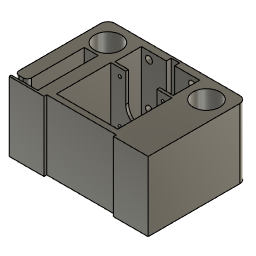
maturita1 v13 asi final (Autodesk Fusion 360 design; units mm, degrees)
Autodesk Fusion 360 part; units mm, degrees
note: some values were not read from the file. Chosen so that the rebuilt part matches the saved one: that a step has no effect. Set by a fixed rule: which sketch regions a step uses.
sketch "Sketch1" plane through (0, 0, 0) normal (0, 0, 1) x (1, 0, 0)
  line L0 (0, 0) -> (25, 0)
  line L1 (25, 0) -> (25, 2)
  line L2 (25, 2) -> (75, 2)
  line L3 (75, 2) -> (75, 0)
  line L4 (75, 0) -> (100, 0)
  line L5 (100, 0) -> (100, 71)
  line L6 (100, 71) -> (0, 71)
  line L7 (0, 71) -> (0, 0)
  dimension "d1" = 50
  dimension "d2" = 25
  dimension "d3" = 71
  constraint coincident L0.start L7.end
  constraint horizontal L0
  constraint perpendicular L0 L1
  constraint perpendicular L1 L2
  constraint perpendicular L2 L3
  constraint perpendicular L3 L4
  constraint perpendicular L4 L5
  constraint perpendicular L5 L6
  constraint perpendicular L0 L7
  measures "d1" distance of L1.end L2.end
  measures "d2" distance of L3.end L4.end
  measures "d3" distance of L4.end L5.end
extrude "Extrude1" add sketch "Sketch1" along normal blind 50
sketch "Sketch2" plane through (0, 0, 50) normal (0, 0, 1) x (-1, 0, 0)
  line L0 (0, -71) -> (0, 0)
  line L1 (0, 0) -> (-25, 0)
  line L2 (-25, 0) -> (-25, -2)
  line L3 (-25, -2) -> (-75, -2)
  line L4 (-75, -2) -> (-75, 0)
  line L5 (-75, 0) -> (-100, 0)
  line L6 (-100, 0) -> (-100, -71)
  line L7 (-100, -71) -> (0, -71)
  line L8 (0, -71) -> (-14.5, -71)
  line L9 (-14.5, -71) -> (-14.5, -56.5)
  circle A0 centre (-14.5, -56.5) radius 9.6
  line L10 (-14.5, -56.5) -> (-85.5, -56.5)
  circle A1 centre (-85.5, -56.5) radius 9.6
  dimension "d6" = 14.5
  dimension "d7" = 14.5
  dimension "d8" = 19.2
  dimension "d9" = 71
  dimension "d10" = 19.2
  constraint coincident L0.start L7.end
  constraint perpendicular L0 L8
  constraint perpendicular L7 L9
  constraint coincident L9.end A0.centre
  constraint perpendicular L9 L10
  constraint coincident L10.end A1.centre
  measures "d6" distance of L0.start L8.end
  measures "d7" distance of L8.end L9.end
  measures "d8" diameter of A0
  measures "d9" distance of L9.end L10.end
  measures "d10" diameter of A1
extrude "Extrude2" cut sketch "Sketch2" against normal up to surface (50 mm away) contours L9 A0 L10 | L9 A0 L10 | A1
fillet "Fillet1" radius 5 2 edges at (100, 71, 25) (0, 71, 25)
sketch "Sketch3" plane through (0, 0, 50) normal (0, 0, 1) x (-1, 0, 0)
  arc A0 (-5, -71) -> (0, -66) centre (-5, -66) ccw
  line L0 (0, -66) -> (0, 0)
  line L1 (0, 0) -> (-25, 0)
  line L2 (-25, 0) -> (-25, -2)
  line L3 (-25, -2) -> (-75, -2)
  line L4 (-75, -2) -> (-75, 0)
  line L5 (-75, 0) -> (-100, 0)
  line L6 (-100, 0) -> (-100, -66)
  arc A1 (-100, -66) -> (-95, -71) centre (-95, -66) ccw
  line L7 (-95, -71) -> (-5, -71)
  circle A2 centre (-14.5, -56.5) radius 9.6
  circle A3 centre (-85.5, -56.5) radius 9.6
  line L8 (-14.5, -66.1) -> (-29, -66.1)
  line L9 (-29, -66.1) -> (-71, -66.1)
  line L10 (-71, -66.1) -> (-71, -47.1)
  line L11 (-71, -47.1) -> (-29, -47.1)
  line L12 (-29, -47.1) -> (-29, -66.1)
  dimension "d22" = 42
  dimension "d23" = 19
  constraint coincident A2 L8.start
  constraint tangent A2 L8
  constraint horizontal L9
  constraint vertical L10
  constraint horizontal L11
  constraint vertical L12
  measures "d22" distance of L8.end L9.end
  measures "d23" distance of L8.end L11.end
extrude "Extrude4" [no effect]
extrude "Extrude5" cut sketch "Sketch3" against normal up to surface (50 mm away) contours L9 L10 L11 L12
sketch "Sketch5" plane through (0, 0, 50) normal (0, 0, 1) x (-1, 0, 0)
  line L0 (-29, -47.1) -> (-29, -66.1)
  line L1 (-29, -66.1) -> (-71, -66.1)
  line L2 (-71, -66.1) -> (-71, -47.1)
  line L3 (-71, -47.1) -> (-29, -47.1)
  arc A0 (-5, -71) -> (0, -66) centre (-5, -66) ccw
  line L4 (0, -66) -> (0, 0)
  line L5 (0, 0) -> (-25, 0)
  line L6 (-25, 0) -> (-25, -2)
  line L7 (-25, -2) -> (-75, -2)
  line L8 (-75, -2) -> (-75, 0)
  line L9 (-75, 0) -> (-100, 0)
  line L10 (-100, 0) -> (-100, -66)
  arc A1 (-100, -66) -> (-95, -71) centre (-95, -66) ccw
  line L11 (-95, -71) -> (-5, -71)
  circle A2 centre (-14.5, -56.5) radius 9.6
  circle A3 centre (-85.5, -56.5) radius 9.6
  line L12 (-50, -2) -> (-28, -2)
  line L13 (-28, -2) -> (-28, -45.1)
  line L14 (-28, -45.1) -> (-72, -45.1)
  line L15 (-72, -45.1) -> (-72, -6.1)
  line L16 (-72, -6.1) -> (-28, -6.1)
  line L17 (-28, -6.1) -> (-28, -45.1)
  line L18 (-50, -6.1) -> (-41, -6.1)
  line L19 (-41, -6.1) -> (-59, -6.1)
  line L20 (-59, -6.1) -> (-59, -18.1)
  line L21 (-59, -18.1) -> (-41, -18.1)
  line L22 (-41, -18.1) -> (-41, -6.1)
  line L23 (-28, -45.1) -> (-38.75, -45.1)
  line L24 (-38.75, -45.1) -> (-61.25, -45.1)
  line L25 (-61.25, -45.1) -> (-61.25, -47.1)
  line L26 (-61.25, -47.1) -> (-38.75, -47.1)
  line L27 (-38.75, -47.1) -> (-38.75, -45.1)
  dimension "d28" = 22
  dimension "d29" = 43.1
  dimension "d30" = 44
  dimension "d31" = 39
  dimension "d32" = 9
  dimension "d33" = 18
  dimension "d34" = 12
  dimension "d35" = 10.75
  dimension "d36" = 22.5
  constraint midpoint L7 L12.start
  constraint parallel L7 L12
  constraint perpendicular L3 L13
  constraint horizontal L14
  constraint vertical L15
  constraint horizontal L16
  constraint vertical L17
  constraint midpoint L16 L18.start
  constraint parallel L16 L18
  constraint horizontal L19
  constraint vertical L20
  constraint horizontal L21
  constraint vertical L22
  constraint perpendicular L17 L23
  constraint horizontal L24
  constraint vertical L25
  constraint horizontal L26
  constraint vertical L27
  measures "d28" distance of L12.start L12.end
  measures "d29" distance of L12.end L13.end
  measures "d30" distance of L13.end L14.end
  measures "d31" distance of L13.end L16.end
  measures "d32" distance of L18.start L18.end
  measures "d33" distance of L18.end L19.end
  measures "d34" distance of L18.end L21.end
  measures "d35" distance of L13.end L23.end
  measures "d36" distance of L23.end L24.end
extrude "Extrude6" cut sketch "Sketch5" against normal up to surface (50 mm away) contours L16 L18 L19 L20 L21 L22
extrude "Extrude7" cut sketch "Sketch5" against normal blind 42 contours L13 L14 L15 L16 L17 L20 L21 L22 L23 L24
extrude "Extrude8" cut sketch "Sketch5" against normal blind 32 contours L3 L14 L24 L25 L26 L27
fillet "Fillet2" radius 11.25 2 edges at (38.75, 46.1, 18) (61.25, 46.1, 18)
sketch "Sketch7" plane through (0, 45.1, 0) normal (0, -1, 0) x (1, 0, 0)
  line L0 (38.75, 29.25) -> (38.75, 50)
  line L1 (38.75, 50) -> (28, 50)
  line L2 (28, 50) -> (28, 8)
  line L3 (28, 8) -> (72, 8)
  line L4 (72, 8) -> (72, 50)
  line L5 (72, 50) -> (61.25, 50)
  line L6 (61.25, 50) -> (61.25, 29.25)
  arc A0 (38.75, 29.25) -> (61.25, 29.25) centre (50, 29.25) ccw
  line L7 (28, 8) -> (34.5, 8)
  line L8 (34.5, 8) -> (34.5, 13.5)
  circle A1 centre (34.5, 13.5) radius 1.1
  dimension "d48" = 6.5
  dimension "d49" = 5.5
  dimension "d50" = 2.2
  constraint coincident L2.end L3.start
  constraint perpendicular L2 L7
  constraint perpendicular L3 L8
  constraint coincident L8.end A1.centre
  measures "d48" distance of L2.end L7.end
  measures "d49" distance of L7.end L8.end
  measures "d50" diameter of A1
extrude "Extrude9" cut sketch "Sketch7" against normal up to surface (25.9 mm away) contours A1
pattern_linear "R-Pattern1" count 2 spacing 31 along (1, 0, 0) count 2 spacing 31 along (0, 0, 1) of "Extrude9"
sketch "Sketch8" plane through (0, 71, 0) normal (0, 1, 0) x (-1, 0, 0)
  circle A0 centre (-65.5, 44.5) radius 1.1
  circle A1 centre (-34.5, 44.5) radius 1.1
  circle A2 centre (-65.5, 13.5) radius 1.1
  circle A3 centre (-34.5, 13.5) radius 1.1
  line L0 (-5, 0) -> (-5, 50)
  line L1 (-5, 50) -> (-95, 50)
  line L2 (-95, 50) -> (-95, 0)
  line L3 (-95, 0) -> (-5, 0)
  circle A4 centre (-65.5, 44.5) radius 2.5
  dimension "d57" = 5
  constraint concentric A0 A4
  measures "d57" diameter of A4
extrude "Extrude10" cut sketch "Sketch8" against normal up to surface (4.9 mm away) contours A4
pattern_linear "R-Pattern2" count 2 spacing 31 along (-1, 0, 0) count 2 spacing 31 along (0, 0, -1) of "Extrude10"
sketch "Sketch9" plane through (0, 0, 50) normal (0, 0, 1) x (-1, 0, 0)
  line L0 (-38.75, -45.1) -> (-38.75, -47.1)
  line L1 (-38.75, -47.1) -> (-29, -47.1)
  line L2 (-29, -47.1) -> (-29, -66.1)
  line L3 (-29, -66.1) -> (-71, -66.1)
  line L4 (-71, -66.1) -> (-71, -47.1)
  line L5 (-71, -47.1) -> (-61.25, -47.1)
  line L6 (-61.25, -47.1) -> (-61.25, -45.1)
  line L7 (-61.25, -45.1) -> (-72, -45.1)
  line L8 (-72, -45.1) -> (-72, -6.1)
  line L9 (-72, -6.1) -> (-28, -6.1)
  line L10 (-28, -6.1) -> (-28, -45.1)
  line L11 (-28, -45.1) -> (-38.75, -45.1)
  circle A0 centre (-85.5, -56.5) radius 9.6
  circle A1 centre (-14.5, -56.5) radius 9.6
  arc A2 (-5, -71) -> (0, -66) centre (-5, -66) ccw
  line L12 (0, -66) -> (0, 0)
  line L13 (0, 0) -> (-25, 0)
  line L14 (-25, 0) -> (-25, -2)
  line L15 (-25, -2) -> (-75, -2)
  line L16 (-75, -2) -> (-75, 0)
  line L17 (-75, 0) -> (-100, 0)
  line L18 (-100, 0) -> (-100, -66)
  arc A3 (-100, -66) -> (-95, -71) centre (-95, -66) ccw
  line L19 (-95, -71) -> (-5, -71)
  line L20 (-50, -66.1) -> (-53, -66.1)
  line L21 (-53, -66.1) -> (-47, -66.1)
  line L22 (-47, -66.1) -> (-47, -69.6)
  line L23 (-47, -69.6) -> (-53, -69.6)
  line L24 (-53, -69.6) -> (-53, -66.1)
  dimension "d64" = 3
  dimension "d65" = 6
  dimension "d66" = 3.5
  constraint midpoint L3 L20.start
  constraint parallel L3 L20
  constraint horizontal L21
  constraint vertical L22
  constraint horizontal L23
  constraint vertical L24
  measures "d64" distance of L20.start L20.end
  measures "d65" distance of L20.end L21.end
  measures "d66" distance of L20.end L23.end
extrude "Extrude11" cut sketch "Sketch9" against normal blind 26.5 contours L3 L20 L21 L22 L23 L24
fillet "Fillet3" radius 3 2 edges at (53, 67.85, 23.5) (47, 67.85, 23.5)
sketch "Sketch10" plane through (0, 0, 50) normal (0, 0, 1) x (-1, 0, 0)
  line L0 (-53, -69.6) -> (-53, -66.1)
  line L1 (-53, -66.1) -> (-71, -66.1)
  line L2 (-71, -66.1) -> (-71, -47.1)
  line L3 (-71, -47.1) -> (-61.25, -47.1)
  line L4 (-61.25, -47.1) -> (-61.25, -45.1)
  line L5 (-61.25, -45.1) -> (-72, -45.1)
  line L6 (-72, -45.1) -> (-72, -6.1)
  line L7 (-72, -6.1) -> (-28, -6.1)
  line L8 (-28, -6.1) -> (-28, -45.1)
  line L9 (-28, -45.1) -> (-38.75, -45.1)
  line L10 (-38.75, -45.1) -> (-38.75, -47.1)
  line L11 (-38.75, -47.1) -> (-29, -47.1)
  line L12 (-29, -47.1) -> (-29, -66.1)
  line L13 (-29, -66.1) -> (-47, -66.1)
  line L14 (-47, -66.1) -> (-47, -69.6)
  line L15 (-47, -69.6) -> (-53, -69.6)
  circle A0 centre (-85.5, -56.5) radius 9.6
  circle A1 centre (-14.5, -56.5) radius 9.6
  arc A2 (-5, -71) -> (0, -66) centre (-5, -66) ccw
  line L16 (0, -66) -> (0, 0)
  line L17 (0, 0) -> (-25, 0)
  line L18 (-25, 0) -> (-25, -2)
  line L19 (-25, -2) -> (-75, -2)
  line L20 (-75, -2) -> (-75, 0)
  line L21 (-75, 0) -> (-100, 0)
  line L22 (-100, 0) -> (-100, -66)
  arc A3 (-100, -66) -> (-95, -71) centre (-95, -66) ccw
  line L23 (-95, -71) -> (-5, -71)
  line L24 (0, 0) -> (-9, 0)
  line L25 (-9, 0) -> (-9, -4)
  line L26 (-9, -4) -> (-19, -4)
  line L27 (-19, -4) -> (-19, -45)
  line L28 (-19, -45) -> (-9, -45)
  line L29 (-9, -45) -> (-9, -4)
  line L30 (-19, -4) -> (0, -4)
  line L31 (0, -4) -> (0, -1.5)
  line L32 (0, -1.5) -> (-19, -1.5)
  line L33 (-19, -1.5) -> (-19, -4)
  dimension "d71" = 9
  dimension "d72" = 4
  dimension "d73" = 10
  dimension "d74" = 41
  dimension "d75" = 19
  dimension "d76" = 2.5
  constraint coincident L16.end L17.start
  constraint perpendicular L8 L24
  constraint perpendicular L24 L25
  constraint horizontal L26
  constraint vertical L27
  constraint horizontal L28
  constraint vertical L29
  constraint horizontal L30
  constraint vertical L31
  constraint horizontal L32
  constraint vertical L33
  measures "d71" distance of L16.end L24.end
  measures "d72" distance of L24.end L25.end
  measures "d73" distance of L25.end L26.end
  measures "d74" distance of L25.end L28.end
  measures "d75" distance of L26.end L30.end
  measures "d76" distance of L26.end L32.end
extrude "Extrude12" cut sketch "Sketch10" against normal blind 16.5 contours L16 L25 L30 L31 L32 | L25 L26 L30 L32 L33 | L26 L27 L28 L29 L30
fillet "Fillet4" radius 3 1 edges at (0, 4, 41.75)
fillet "Fillet5" radius 3 1 edges at (0, 4.25, 33.5)
fillet "Fillet6" radius 3 1 edges at (9, 4, 41.75)
sketch "Sketch11" plane through (0, 71, 0) normal (0, 1, 0) x (-1, 0, 0)
  circle A0 centre (-65.5, 13.5) radius 2.5
  line L0 (-5, 0) -> (-5, 50)
  line L1 (-5, 50) -> (-95, 50)
  line L2 (-95, 50) -> (-95, 0)
  line L3 (-95, 0) -> (-5, 0)
  circle A1 centre (-65.5, 44.5) radius 2.5
  circle A2 centre (-34.5, 44.5) radius 2.5
  circle A3 centre (-34.5, 13.5) radius 2.5
  line L4 (-95, 50) -> (-85.25, 50)
  line L5 (-85.25, 50) -> (-85.25, 25)
  circle A4 centre (-85.25, 25) radius 2.5
  line L6 (-85.25, 25) -> (-14.75, 25)
  circle A5 centre (-14.75, 25) radius 2.5
  dimension "d85" = 9.75
  dimension "d86" = 25
  dimension "d87" = 5
  dimension "d88" = 70.5
  dimension "d89" = 5
  constraint coincident L1.end L2.start
  constraint perpendicular L2 L4
  constraint perpendicular L3 L5
  constraint coincident L5.end A4.centre
  constraint perpendicular L5 L6
  constraint coincident L6.end A5.centre
  measures "d85" distance of L1.end L4.end
  measures "d86" distance of L4.end L5.end
  measures "d87" diameter of A4
  measures "d88" distance of L5.end L6.end
  measures "d89" diameter of A5
extrude "Extrude13" cut sketch "Sketch11" against normal blind 6 contours L5 A4 L6 | L5 A4 L6 | A5
fillet "Fillet7" radius 2 2 edges at (87.5808, 71, 25.904) (17.0808, 71, 25.904)
equation "d29 = 45.100 mm - 2 mm"
equation "d35 = ( ( 44 - 22.5 ) / 2 ) * 1 mm"
equation "d67 = -21 mm - 5.5 mm"
equation "d71 = ( ( 28 - 10 ) / 2 ) * 1 mm"
equation "d85 = ( 19.5 / 2 ) * 1 mm"
equation "d88 = 100 mm - 5 mm - 9.75 mm - 5 mm - 9.75 mm"
